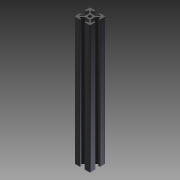
# Autodesk Inventor part: 2020 extrusion 165mm short cross
Saved by Autodesk Inventor 2014 SP1 (Build 180222100, 222)
## iProperties
Category: PARTsolutions
Company: MISUMI
Created: 2014-09-21
Part Number: 2020 extrusion 165mm short cross
Catalog Web Link: www.cadenas.de
Description: HFS5-2020, HFSB5-2020, CAF5-2020, HFSY5-2020, HFSF5-2020, HFSFB5-2020, HFST5-2020, HFSTB5-2020, HFSH5-2020, HFSC5-2020-HFS5 Series Aluminum Extrusions 20 Square -1 Slot-
Vendor: MISUMI
Document SubType Name: Modeling
Designer: psAdmin
Manufacturer: MISUMI
Mass: 72.7919 g
Surface Area: 694.63 cm^2
Volume: 72.7919 cm^3
Density: 1 g/cm^3
Material: Generic
Appearance: PSOLRGB-175-175-175
PSOL_IDENT_0: {\\10.0.0.236\data_v8\23d-libs\misumi\metric\38_al_extrusions_blackets\5\hfs5_2020.prj},524 {VTYP=3D
PSOL_IDENT_1: },{NB=CAF5-2020-400},{LINA=CAF5-2020-400},{NN=HFS5-2020, HFSB5-2020, CAF5-2020, HFSY5-2020, HFSF5-20
PSOL_IDENT_2: 20, HFSFB5-2020, HFST5-2020, HFSTB5-2020, HFSH5-2020, HFSC5-2020},{DATE=26.08.2014 05:22:23},{GEOMDA
PSOL_IDENT_3: TE=27.10.2011 00:00:00},{VERSION=},{LINEID=40},{LINESUBID=-1},{WBVAR=L,ALT1,ALT2,ALT3,CPS,CDSL,CDSR,
PSOL_IDENT_4: ALT4,HPS,NOHL,HDL,NOHR,HDR,ALT41,ALT42,ALT5H,NOMH5H,AH,BH,CH,DH,EH,ALT5V,NOMH5V,AV,BV,CV,DV,EV,ALT5P
PSOL_IDENT_5: ,NOMH5P,AP,BP,CP,DP,EP,ALT6V,ALT6H,Z,NOMH6V,NOMH6H,XA,XB,XC,XD,XE,YA,YB,YC,YD,YE,ALT7,HPS7,HDL7,HDR7
PSOL_IDENT_6: ,ALT8T,HQ,JLP}  {NB=CAF5-2020-400},{LINA=CAF5-2020-400},{KT=DUMMY},{PN=CAF5-2020-400},{TPS=CAF5-2020
PSOL_IDENT_7: },{MAT=A6N01SS-T5 Aluminum Alloy or 6005A-T5 Aluminum Alloy},{ST=Clear Coating (Clear Anodize + Clea
PSOL_IDENT_8: r Painting)},{FRMW=20},{FRMH=20},{L=400},{MASS=0.5},{SA=183},{LX=0.742x10^4},{LY=0.742x10^4},{ALT1=}
PSOL_IDENT_9: ,{ALT2=},{ALT2ALG= '', 'w/o SC (High Precision Cut)', '-SC', 'with SC (High Precision Cut)' },{ALT3=
PSOL_IDENT_10: },{ALT3ALG= '','w/o 45 Degree Cut','1','with 45 Degree Cut' },{CPS=},{CPSALG= '','N/A' },{CDSL=},{CD
PSOL_IDENT_11: SLALG= '','N/A' },{CDSR=},{CDSRALG= '','N/A' },{ALT3PN=},{ALT4=},{ALT4ALG= '','w/o Fastening Locatio
PSOL_IDENT_12: n Wrench Access Hole Alterations','1','with Fastening Location Wrench Access Hole Alterations' },{HL=
PSOL_IDENT_13: 10},{HR=10},{J=20},{K=20},{DD4=7.35},{HPS=},{HPSALG= '','N/A' },{NOHL=},{NOHLALG= '','N/A' },{HDL=},
PSOL_IDENT_14: {HDLALG= '','N/A' },{NOHR=},{NOHRALG= '','N/A' },{HDR=},{HDRALG= '','N/A' },{ALT41=},{ALT41ALG= '','
PSOL_IDENT_15: N/A' },{ALT42=},{ALT42ALG= '','N/A' },{ALT4PN=},{ALT5H=},{ALT5HALG= '','w/o Location Specified Wrenc
PSOL_IDENT_16: h Access Hole Alteratons (Horizontal)','1','with Location Specified Wrench Access Hole Alteratons (H
PSOL_IDENT_17: orizontal)' },{NOMH5H=0},{NOMH5HMAX=5},{NOMH5HALG=[0]},{AH=0},{AHMIN=7},{AHMAX=402.35},{AHALG=[0]},{
PSOL_IDENT_18: BH=0},{BHMIN=10},{BHMAX=411.7},{BHALG=[0]},{CH=0},{CHMIN=10},{CHMAX=421.05},{CHALG=[0]},{DH=0},{DHMI
PSOL_IDENT_19: N=10},{DHMAX=430.4},{DHALG=[0]},{EH=0},{EHMIN=10},{EHMAX=393},{EHALG=[0]},{ALT5V=},{ALT5VALG= '','w/
PSOL_IDENT_20: o Location Specified Wrench Access Hole Alteratons (Vertical)','1','with Location Specified Wrench A
PSOL_IDENT_21: ccess Hole Alteratons (Vertical)' },{NOMH5V=0},{NOMH5VMAX=5},{NOMH5VALG=[0]},{AV=0},{AVMIN=7},{AVMAX=
PSOL_IDENT_22: 402.35},{AVALG=[0]},{BV=0},{BVMIN=10},{BVMAX=411.7},{BVALG=[0]},{CV=0},{CVMIN=10},{CVMAX=421.05},{CV
PSOL_IDENT_23: ALG=[0]},{DV=0},{DVMIN=10},{DVMAX=430.4},{DVALG=[0]},{EV=0},{EVMIN=10},{EVMAX=393},{EVALG=[0]},{ALT5
PSOL_IDENT_24: P=},{ALT5PALG= '','w/o Location Specified Wrench Access Hole Alteratons (Crisscross)','1','with Loca
PSOL_IDENT_25: tion Specified Wrench Access Hole Alteratons (Crisscross)' },{NOMH5P=0},{NOMH5PMAX=5},{NOMH5PALG=[0]
PSOL_IDENT_26: },{AP=0},{APMIN=7},{APMAX=402.35},{APALG=[0]},{BP=0},{BPMIN=10},{BPMAX=411.7},{BPALG=[0]},{CP=0},{CP
PSOL_IDENT_27: MIN=10},{CPMAX=421.05},{CPALG=[0]},{DP=0},{DPMIN=10},{DPMAX=430.4},{DPALG=[0]},{EP=0},{EPMIN=10},{EP
PSOL_IDENT_28: MAX=393},{EPALG=[0]},{ALT5HPN=},{ALT5VPN=},{ALT5PPN=},{ALT5PN=},{ALT6V=},{ALT6VALG= '','w/o Counterb
PSOL_IDENT_29: ore Hole in Specified Position (Vertical)','1','with Counterbore Hole in Specified Position (Vertica
PSOL_IDENT_30: l)' },{ALT6H=},{ALT6HALG= '','w/o Counterbore Hole in Specified Position (Horizontal)','1','with Cou
PSOL_IDENT_31: nterbore Hole in Specified Position (Horizontal)' },{Z=},{ZALG= '','N/A' },{NOMH6V=0},{NOMH6VMAX=5},
PSOL_IDENT_32: {NOMH6VALG=[0]},{NOMH6H=0},{NOMH6HMAX=5},{NOMH6HALG=[0]},{DD6=13.0},{DD16=19.0},{XA=0},{XAMIN=7},{XA
PSOL_IDENT_33: MAX=414},{XAALG=[0]},{XB=0},{XBMIN=16},{XBMAX=435},{XBALG=[0]},{XC=0},{XCMIN=16},{XCMAX=456},{XCALG=
PSOL_IDENT_34: [0]},{XD=0},{XDMIN=16},{XDMAX=477},{XDALG=[0]},{XE=0},{XEMIN=16},{XEMAX=393},{XEALG=[0]},{YA=0},{YAM
PSOL_IDENT_35: IN=7},{YAMAX=414},{YAALG=[0]},{YB=0},{YBMIN=16},{YBMAX=435},{YBALG=[0]},{YC=0},{YCMIN=16},{YCMAX=456
PSOL_IDENT_36: },{YCALG=[0]},{YD=0},{YDMIN=16},{YDMAX=477},{YDALG=[0]},{YE=0},{YEMIN=16},{YEMAX=393},{YEALG=[0]},{A
PSOL_IDENT_37: LT6XPN=},{ALT6YPN=},{ALT6PN=},{ALT7=},{ALT7ALG= '','w/o M Type Hole Alteration','1','with M Type Hol
PSOL_IDENT_38: e Alteration' },{HPS7=},{HPS7ALG= '','N/A' },{HDL7=},{HDL7ALG= '','N/A' },{HDR7=},{HDR7ALG= '','N/A'
PSOL_IDENT_39: },{H7=10},{D7=7.1},{ALT7PN=},{ALT8T=},{ALT8TALG= '','w/o L Type Hole Alteration (Top)','1','with L
PSOL_IDENT_40: Type Hole Alteration (Top)' },{HQ=0},{HQALG=0},{JLP=0},{JLPMIN=12},{JLPMAX=0},{JLPALG=[0]},{L1=0},{D
PSOL_IDENT_41: 8=7.1},{ALT8PN=}
SUPPLIER: MISUMI
ARTICLENO: CAF5-2020-400
BOMINFO: CAF5-2020-400
CREATOR: CADENAS GmbH
Title: CAF5-2020-400
Author: Cadenas PARTsolutions
Comments: HFS5 Series Aluminum Extrusions 20 Square -1 Slot-
Autodesk Inventor part; units mm, degrees
sketch "Sketch_1" plane through (0, 0, 0) normal (0, 0, 1) x (1, 0, 0)
  line L0 (-10, 9) -> (-10, 3.3)
  arc A0 (-10, 3.3) -> (-9.7, 3) centre (-9.7, 3.3) ccw
  line L1 (-9.7, 3) -> (-8, 3)
  line L2 (-8, 3) -> (-8, 6)
  line L3 (-8, 6) -> (-7.0607, 6)
  line L4 (-7.0607, 6) -> (-4, 2.9393)
  line L5 (-4, 2.9393) -> (-4, 0.5196)
  line L6 (-4, 0.5196) -> (-3.7, 0)
  line L7 (-3.7, 0) -> (-4, -0.5196)
  line L8 (-4, -0.5196) -> (-4, -2.9393)
  line L9 (-4, -2.9393) -> (-7.0607, -6)
  line L10 (-7.0607, -6) -> (-8, -6)
  line L11 (-8, -6) -> (-8, -3)
  line L12 (-8, -3) -> (-9.7, -3)
  arc A1 (-9.7, -3) -> (-10, -3.3) centre (-9.7, -3.3) ccw
  line L13 (-10, -3.3) -> (-10, -9)
  arc A2 (-10, -9) -> (-9, -10) centre (-9, -9) ccw
  line L14 (-9, -10) -> (-3.3, -10)
  arc A3 (-3.3, -10) -> (-3, -9.7) centre (-3.3, -9.7) ccw
  line L15 (-3, -9.7) -> (-3, -8)
  line L16 (-3, -8) -> (-6, -8)
  line L17 (-6, -8) -> (-6, -7.0607)
  line L18 (-6, -7.0607) -> (-2.9393, -4)
  line L19 (-2.9393, -4) -> (-0.5196, -4)
  line L20 (-0.5196, -4) -> (0, -3.7)
  line L21 (0, -3.7) -> (0.5196, -4)
  line L22 (0.5196, -4) -> (2.9393, -4)
  line L23 (2.9393, -4) -> (6, -7.0607)
  line L24 (6, -7.0607) -> (6, -8)
  line L25 (6, -8) -> (3, -8)
  line L26 (3, -8) -> (3, -9.7)
  arc A4 (3, -9.7) -> (3.3, -10) centre (3.3, -9.7) ccw
  line L27 (3.3, -10) -> (9, -10)
  arc A5 (9, -10) -> (10, -9) centre (9, -9) ccw
  line L28 (10, -9) -> (10, -3.3)
  arc A6 (10, -3.3) -> (9.7, -3) centre (9.7, -3.3) ccw
  line L29 (9.7, -3) -> (8, -3)
  line L30 (8, -3) -> (8, -6)
  line L31 (8, -6) -> (7.0606, -6)
  line L32 (7.0606, -6) -> (4, -2.9393)
  line L33 (4, -2.9393) -> (4, -0.5196)
  line L34 (4, -0.5196) -> (3.7, 0)
  line L35 (3.7, 0) -> (4, 0.5196)
  line L36 (4, 0.5196) -> (4, 2.9393)
  line L37 (4, 2.9393) -> (7.0607, 6)
  line L38 (7.0607, 6) -> (8, 6)
  line L39 (8, 6) -> (8, 3)
  line L40 (8, 3) -> (9.7, 3)
  arc A7 (9.7, 3) -> (10, 3.3) centre (9.7, 3.3) ccw
  line L41 (10, 3.3) -> (10, 9)
  arc A8 (10, 9) -> (9, 10) centre (9, 9) ccw
  line L42 (9, 10) -> (3.3, 10)
  arc A9 (3.3, 10) -> (3, 9.7) centre (3.3, 9.7) ccw
  line L43 (3, 9.7) -> (3, 8)
  line L44 (3, 8) -> (6, 8)
  line L45 (6, 8) -> (6, 7.0607)
  line L46 (6, 7.0607) -> (2.9393, 4)
  line L47 (2.9393, 4) -> (0.5196, 4)
  line L48 (0.5196, 4) -> (0, 3.7)
  line L49 (0, 3.7) -> (-0.5196, 4)
  line L50 (-0.5196, 4) -> (-2.9394, 4)
  line L51 (-2.9394, 4) -> (-6, 7.0606)
  line L52 (-6, 7.0606) -> (-6, 8)
  line L53 (-6, 8) -> (-3, 8)
  line L54 (-3, 8) -> (-3, 9.7)
  arc A10 (-3, 9.7) -> (-3.3, 10) centre (-3.3, 9.7) ccw
  line L55 (-3.3, 10) -> (-9, 10)
  arc A11 (-9, 10) -> (-10, 9) centre (-9, 9) ccw
  constraints: 112 end point, 24 point on circle, 12 centre point
extrude "Extrusion1" add sketch "Sketch_1" against normal blind 165
sketch "Sketch_2" plane through (0, 0, 0) normal (1, 0, 0) x (0, 0, -1)
  line L0 (400, 0) -> (0, 0)
  line L1 (0, 0) -> (0, 2.1)
  line L2 (0, 2.1) -> (400, 2.1)
  line L3 (400, 2.1) -> (400, 0)
  line L4 (400, 0) -> (0, 0)
  constraints: 10 end point
revolve "Revolution1" cut sketch "Sketch_2" angle 360 about axis through (0, 0, -400) along (0, 0, -1)
ref_plane "C1_XY" through (0, 0, 0) normal (0, 0, 1) x (1, 0, 0)
ref_plane "C1_YZ" through (0, 0, 0) normal (1, 0, 0) x (0, 1, 0)
ref_plane "C1_ZX" through (0, 0, 0) normal (0, 1, 0) x (0, 0, 1)
body "Solid1"
